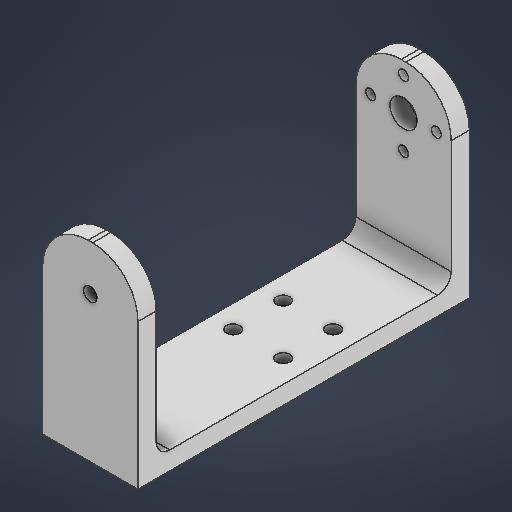
# Autodesk Inventor part: L1
Saved by Autodesk Inventor 2026.1 (Build 301233000, 233)
## iProperties
Created: 2025-09-17
Part Number: L1
Material: Generic
Document SubType Name: Modeling
Designer: emanuel
Density: 1 g/cm^3
Appearance: Default
Author: emanuel
Autodesk Inventor part; units mm, degrees
ref_plane "YZ Plane" through (0, 0, 0) normal (1, 0, 0) x (0, 1, 0)
ref_plane "XZ Plane" through (0, 0, 0) normal (0, 1, 0) x (-1, 0, 0)
ref_plane "XY Plane" through (0, 0, 0) normal (0, 0, 1) x (1, 0, 0)
sketch "Sketch1" plane through (0, 0, 0) normal (1, 0, 0) x (0, 1, 0)
  line L0 (0, 0) -> (0, -36)
  line L1 (0, -36) -> (38, -36)
  line L2 (0, 0) -> (-4, 0)
  line L3 (-4, 0) -> (-4, -40)
  line L4 (-4, -40) -> (38, -40)
  line L5 (38, -40) -> (38, -36)
  line L6 (0, 0) -> (-4, 0)
  line L7 (-4, 0) -> (-4, 29)
  line L8 (-4, 29) -> (0, 29)
  line L9 (0, 29) -> (0, 0)
  line L10 (-4, 29) -> (38, 29)
  line L11 (38, 29) -> (38, 33)
  line L12 (38, 33) -> (-4, 33)
  line L13 (-4, 33) -> (-4, 29)
  point P0 (0, 29)
  dimension "d0" = 36
  dimension "d1" = 38
  dimension "d2" = 4
  dimension "d3" = 40
  dimension "d28" = 29
  dimension "d29" = 42
  dimension "d30" = 4
  constraints: 28 end point, 6 perpendicular, 4 parallel, 3 horizontal, 1 vertical
  measures "d0" distance of L0.start L0.end
  measures "d1" distance of L0.end L1.end
  measures "d2" distance of L0.start L2.end
  measures "d3" distance of L2.end L3.end
  measures "d28" distance of L6.end L7.end
  measures "d29" distance of L12.end L11.end
  measures "d30" distance of L11.end L10.end
extrude "Extrusion1" add sketch "Sketch1" along normal blind 21 contours L0 L1 L5 L4 L3 L2
fillet "Fillet1" radius 10 2 edges at (21, 38, -38) (0, 38, -38)
sketch "Sketch2" plane through (0, 0, -36) normal (0, 0, 1) x (1, 0, 0)
  arc A0 (10, 38) -> (0, 28) centre (10, 28) ccw projected
  line L0 (0, 28) -> (21, 28)
  line L1 (0, 28) -> (0, 0) projected
  line L2 (0, 28) -> (10.5, 28)
  circle A1 centre (10.5, 28) radius 8
  circle A2 centre (10.5, 28) radius 6.5
  line L3 (4, 28) -> (2.5, 28)
  circle A3 centre (3.25, 28) radius 1.1
  line L4 (17, 28) -> (18.5, 28)
  circle A4 centre (17.75, 28) radius 1.1
  line L5 (10.5, 28) -> (10.5, 36)
  line L6 (10.5, 28) -> (10.5, 20)
  line L7 (10.5, 36) -> (10.5, 34.5)
  line L8 (10.5, 20) -> (10.5, 21.5)
  circle A5 centre (10.5, 35.25) radius 1.1
  circle A6 centre (10.5, 20.75) radius 1.1
  circle A7 centre (10.5, 28) radius 3
  dimension "d7" = 10.5
  dimension "d8" = 16
  dimension "d9" = 13
  dimension "d10" = 2.2
  dimension "d11" = 2.2
  dimension "d12" = 2.2
  dimension "d13" = 2.2
  dimension "d14" = 6
  constraints: 16 end point, 8 point on circle, 7 centre point, 7 point on line, 5 midpoint, 3 coincident, 1 vertical
  measures "d7" distance of L0.start L2.end
  measures "d8" diameter of A1
  measures "d9" diameter of A2
  measures "d10" diameter of A3
  measures "d11" diameter of A4
  measures "d12" diameter of A5
  measures "d13" diameter of A6
  measures "d14" diameter of A7
extrude "Extrusion2" cut sketch "Sketch2" against normal blind 21 contours A2 A3 A1 L0 | A2 A3 L0 | L0 A1 A3 A2 | L0 A3 A2 | A1 A3 L0 | L0 A3 A1 | A7 L5 L0 | L0 L6 A7 | A5 A1 L5 A2 | A2 L5 A5 | A6 L6 A2 | A2 L6 A1 A6 | A5 A1 | A1 A6 | L5 A7 L0 | L0 A7 L6 | L5 A1 A5 A2 | A2 A5 L5 | L6 A6 A2 | A2 A6 A1 L6 | A4 L0 A1 | A1 L0 A2 A4 | A4 A2 L0 A1 | A1 L0 A4 | A4 A2 L0 | L0 A2 A4
fillet "Fillet2" radius 3 1 edges at (10.5, 0, -36)
extrude "Extrusion4" add sketch "Sketch1" along normal up to surface (21 mm away) contours L2 L7 L8 L9 | L8 L13 L12 L11 L10
fillet "Fillet3" radius 10 2 edges at (0, 38, 31) (21, 38, 31)
fillet "Fillet4" radius 3 1 edges at (10.5, 0, 29)
sketch "Sketch4" plane through (11, 38, 29) normal (0, 0, -1) x (-1, 0, 0)
  line L0 (-10, -10) -> (0.5, -10)
  circle A0 centre (0.5, -10) radius 1.5
  point P0 (11, -38)
  dimension "d35" = 10.5
  dimension "d36" = 3
  constraints: 2 end point, 1 centre point, 1 coincident, 1 horizontal
  measures "d35" distance of L0.start L0.end
  measures "d36" diameter of A0
extrude "Extrusion5" cut sketch "Sketch4" against normal blind 10
sketch "Sketch5" plane through (0, 0, -33) normal (0, 1, 0) x (1, 0, 0)
  line L0 (0, -59) -> (0, -62) projected
  line L1 (0, -59) -> (0, -29)
  line L2 (0, 0) -> (0, -59) projected
  line L3 (0, -29) -> (5, -29)
  line L4 (21, 0) -> (21, -59) projected
  line L5 (5, -29) -> (16, -29)
  line L6 (5, -29) -> (16, -29)
  line L7 (16, -29) -> (16, -18)
  line L8 (16, -18) -> (5, -18)
  line L9 (5, -18) -> (5, -29)
  circle A0 centre (5, -18) radius 1.5
  circle A1 centre (16, -18) radius 1.5
  circle A2 centre (5, -29) radius 1.5
  circle A3 centre (16, -29) radius 1.5
  point P0 (0, -33)
  dimension "d40" = 30
  dimension "d41" = 5
  dimension "d42" = 11
  dimension "d43" = 11
  dimension "d44" = 11
  dimension "d45" = 3
  dimension "d46" = 3
  dimension "d47" = 3
  dimension "d48" = 3
  constraints: 14 end point, 4 centre point, 4 coincident, 2 parallel, 2 perpendicular, 2 point on line, 1 horizontal
  measures "d40" distance of L0.start L1.end
  measures "d41" distance of L1.end L3.end
  measures "d42" distance of L3.end L5.end
  measures "d43" distance of L8.end L7.end
  measures "d44" distance of L7.end L6.end
  measures "d45" diameter of A0
  measures "d46" diameter of A1
  measures "d47" diameter of A2
  measures "d48" diameter of A3
extrude "Extrusion6" cut sketch "Sketch5" against normal blind 10 contours A2 L9 L3 | L3 L5 A2 | L9 A2 L5 | A0 L8 L9 | L9 L8 A0 | A3 L7 L5 | L5 L7 A3 | A1 L7 L8 | L8 L7 A1
body "Solid1"
